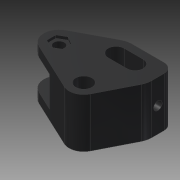
# Autodesk Inventor part: Y_tensioner
Saved by Autodesk Inventor 2013 (Build 170138000, 138)
## iProperties
Created: 2014-01-31
Part Number: Y_tensioner
Material: Ogólny
Document SubType Name: Modeling
Designer: Piotr
Density: 1 g/cm^3
Author: Piotr
Autodesk Inventor part; units mm, degrees
ref_plane "YZ Plane" through (0, 0, 0) normal (1, 0, 0) x (0, 1, 0)
ref_plane "XZ Plane" through (0, 0, 0) normal (0, 1, 0) x (-1, 0, 0)
sketch "Szkic1" plane through (0, 0, 0) normal (0, 0, 1) x (1, 0, 0)
  circle A0 centre (0, 0) radius 4.25
  line L0 (0, 0) -> (0, 22) construction
  line L1 (-5, 22) -> (5, 22) construction
  line L2 (-5, 17.75) -> (5, 17.75)
  arc A1 (5, 17.75) -> (5, 26.25) centre (5, 22) ccw
  line L3 (5, 26.25) -> (-5, 26.25)
  arc A2 (-5, 26.25) -> (-5, 17.75) centre (-5, 22) ccw
  circle A3 centre (-25, 12) radius 8 construction
  line L4 (-5, 22) -> (-25, 22) construction
  line L5 (-25, 22) -> (-25, 12) construction
  circle A4 centre (-25, 12) radius 2.75
  line L6 (-9.6516, 29.1023) -> (-28.7213, 19.0818)
  arc A5 (-28.7213, 19.0818) -> (-28.3967, 4.7569) centre (-25, 12) ccw
  line L7 (-28.3967, 4.7569) -> (-3.2905, -7.0168)
  arc A6 (-3.2905, -7.0168) -> (6.9098, -3.5096) centre (0, 0) ccw
  line L8 (6.9098, -3.5096) -> (15.9158, 14.2214)
  arc A7 (15.9158, 14.2214) -> (17, 18.75) centre (7, 18.75) ccw
  line L9 (17, 18.75) -> (17, 25.25)
  arc A8 (17, 25.25) -> (12, 30.25) centre (12, 25.25) ccw
  line L10 (12, 30.25) -> (-5, 30.25)
  arc A9 (-5, 30.25) -> (-9.6516, 29.1023) centre (-5, 20.25) ccw
  line L11 (-25, 16.7343) -> (-20.9, 14.3671) construction
  line L12 (-20.9, 14.3671) -> (-20.9, 9.6329) construction
  line L13 (-20.9, 9.6329) -> (-25, 7.2657) construction
  line L14 (-25, 7.2657) -> (-29.1, 9.6329) construction
  line L15 (-29.1, 9.6329) -> (-29.1, 14.3671) construction
  line L16 (-29.1, 14.3671) -> (-25, 16.7343) construction
  line L17 (-5, 22) -> (-5, 30.25) construction
  circle A10 centre (-25, 12) radius 14 construction
  arc A11 (-17.9946, -0.1212) -> (-18.5508, 24.4261) centre (-25, 12) ccw
  dimension "d16" = 28
  dimension "d0" = 8.5
  dimension "d1" = 22
  dimension "d2" = 10
  dimension "d3" = 4.25
  dimension "d4" = 16
  dimension "d5" = 10
  dimension "d6" = 20
  dimension "d7" = 5.5
  dimension "d8" = 12
  dimension "d9" = 4
  dimension "d10" = 7.75
  dimension "d11" = 8.2
  dimension "d12" = 8
  dimension "d13" = 5
  dimension "d14" = 10
  dimension "d15" = 10
  constraints: 36 end point, 16 point on circle, 14 tangent, 11 centre point, 9 coincident, 4 parallel, 4 perpendicular, 3 point on line, 1 midpoint, 1 symmetric about line, 1 vertical, 16 other
  measures "d0" diameter of A0
  measures "d1" distance of L0.end L0.start
  measures "d2" distance of L1.start L1.end
  measures "d3" radius of A1
  measures "d4" diameter of A3
  measures "d5" distance from line of L4 L5.end
  measures "d6" distance of L4.start L4.end
  measures "d7" diameter of A4
  measures "d8" distance from line of L1.end L9
  measures "d9" distance between parallel lines of L10 L3
  measures "d10" radius of A6
  measures "d11" distance between parallel lines of L11 L14
  measures "d12" radius of A5
  measures "d13" radius of A8
  measures "d14" radius of A7
  measures "d15" radius of A9
extrude "Wyciągnięcie proste1" add sketch "Szkic1" along normal mid plane 26
extrude "Wyciągnięcie proste2" cut sketch "Szkic1" along normal mid plane 16 contours A11 L7 A5 L6
sketch "Szkic2" plane through (0, 0, 13) normal (0, 0, 1) x (1, 0, 0)
  circle A0 centre (-25, 12) radius 2.75 projected
  line L0 (-29.1, 14.3671) -> (-25, 16.7343) projected
  line L1 (-29.1, 9.6329) -> (-29.1, 14.3671) projected
  line L2 (-25, 7.2657) -> (-29.1, 9.6329) projected
  line L3 (-20.9, 9.6329) -> (-25, 7.2657) projected
  line L4 (-20.9, 14.3671) -> (-20.9, 9.6329) projected
  line L5 (-25, 16.7343) -> (-20.9, 14.3671) projected
extrude "Wyciągnięcie proste3" cut sketch "Szkic2" against normal blind 1.5
sketch "Szkic3" plane through (17, 18.75, 13) normal (1, 0, 0) x (0, 0, -1)
  line L0 (26, 6.5) -> (0, 6.5) projected
  line L1 (0, 0) -> (26, 6.5) construction
  line L2 (0, 6.5) -> (26, 0) construction
  circle A0 centre (13, 3.25) radius 2.25
  line L3 (13, 3.25) -> (13, 11.5) construction
  line L4 (10.9215, 6.85) -> (15.0785, 6.85)
  line L5 (15.0785, 6.85) -> (17.1569, 3.25)
  line L6 (17.1569, 3.25) -> (15.0785, -0.35)
  line L7 (15.0785, -0.35) -> (10.9215, -0.35)
  line L8 (10.9215, -0.35) -> (8.8431, 3.25)
  line L9 (8.8431, 3.25) -> (10.9215, 6.85)
  line L10 (26, 11.5) -> (0, 11.5) projected
  line L11 (26, 11.5) -> (0, 11.5) projected
  point P0 (13, -18.75)
  point P1 (13, 6.85)
  dimension "d23" = 4.5
  dimension "d24" = 7.2
  constraints: 18 end point, 3 midpoint, 1 centre point, 1 coincident, 1 perpendicular, 1 point on line, 13 other
  measures "d23" diameter of A0
  measures "d24" distance between parallel lines of L5 L8
ref_plane "Płaszczyzna konstrukcyjna1" through (13, 18.75, 13) normal (1, 0, 0) x (0, 0, -1)
extrude "Wyciągnięcie proste4" cut sketch "Szkic3" against normal up to next contours A0
sketch "Szkic4" plane through (13, 18.75, 13) normal (1, 0, 0) x (0, 0, -1)
  line L0 (10.9215, -0.35) -> (8.8431, 3.25) projected
  line L1 (15.0785, -0.35) -> (10.9215, -0.35) projected
  line L2 (17.1569, 3.25) -> (15.0785, -0.35) projected
  line L3 (15.0785, 6.85) -> (17.1569, 3.25) projected
  line L4 (10.9215, 6.85) -> (15.0785, 6.85) projected
  line L5 (8.8431, 3.25) -> (10.9215, 6.85) projected
  point P0 (13, -18.75)
extrude "Wyciągnięcie proste5" cut sketch "Szkic4" against normal up to surface
